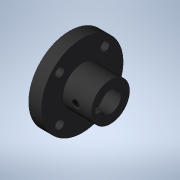
# Autodesk Inventor part: STHRANG8-MB_ss
Saved by Autodesk Inventor 2021 (Build 250183000, 183)
## iProperties
Created: 2025-08-06
Part Number: STHRANG8-MB_ss
Material: Generic
Catalog Web Link: www.cadenas.de
Description: STHRBNG, STHRNG, SSTHRNG, STHRANG_SS-Shaft Supports - with Damper - Key Groove - Round Flange
Vendor: MISUMI
Document SubType Name: Modeling
Designer: psAdmin
Manufacturer: MISUMI
Mass: 4.85232 g
Surface Area: 31.4741 cm^2
Volume: 4.85232 cm^3
Density: 1 g/cm^3
Appearance: PSOLRGB-175-175-175
Category: PARTsolutions
Company: MISUMI
Title: STHRANG8-MB
Author: Cadenas PARTsolutions
Comments: Shaft Supports - with Damper - Key Groove - Round Flange
PSOL_IDENT_0: {$CADENAS_DATA/23d-libs/misumi/metric/02_shaft_supports/sthrbng/sthrbng.prj},207 {VTYP=3D},{NB=STHRA
PSOL_IDENT_1: NG8-MB_ss},{LINA=STHRANG8-MB},{NN=STHRBNG, STHRNG, SSTHRNG, STHRANG_SS},{DATE=18.02.2024 15:03:40},{
PSOL_IDENT_2: GEOMDATE=16.02.2024 10:05:26},{VERSION=},{LINEID=190},{WBVAR=MAT,ST,ALT1},{WBNUMERIC=}  {NB=STHRANG8
PSOL_IDENT_3: -MB_ss},{LINA=STHRANG8-MB},{KT=DUMMY},{PN=STHRANG8-MB},{TYPE=STHRANG},{MAT=5052},{ST=-},{D=8},{DTOL=
PSOL_IDENT_4: +0.015/0},{N=3.5},{L=16},{S=0},{L1=0},{D1=15},{H=32},{T=5},{LL=10},{M=M3},{THMD=3},{THDMIN=2.459},{P=
PSOL_IDENT_5: 25},{K=0},{W=15},{P1=25},{F=0},{DD1=3.5},{ST0='-','-'},{BB=3},{BBTOL=+0.013/-0.013},{TT=1.8},{TTTOL=
PSOL_IDENT_6: +0.1/0},{ALT1=MB},{MBM=M3},{ML=3},{ALT1PN=-MB},{MATALG= '1045', 'S45C Equivalent', '304', 'SUS304','
PSOL_IDENT_7: 5052','5052 Aluminum Alloy' }
NB: STHRANG8-MB_ss
NN: STHRBNG, STHRNG, SSTHRNG, STHRANG_SS
NT: Shaft Supports - with Damper - Key Groove - Round Flange
NBSYN: $PN._ss
LINA: STHRANG8-MB
CATALOG: Misumi
PN: STHRANG8-MB
MAT: 5052 Aluminum Alloy
ST: -
D: 8
DTOL: +0.015/0
N: 3.5
L: 16
S: 0
L1: 0
D1: 15
H: 32
T: 5
LL: 10
M: M3
P: 25
W: 15
P1: 25
F: 0
DD1: 3.5
BB: 3
BBTOL: +0.013/-0.013
TT: 1.8
TTTOL: +0.1/0
MBM: M3
ML: 3
SUPPLIER: MISUMI
ARTICLENO: STHRANG8-MB_ss
BOMINFO: STHRANG8-MB
CREATOR: CADENAS GmbH
Autodesk Inventor part; units mm, degrees
sketch "Sketch_1" plane through (0, 0, 0) normal (0, 0, 1) x (1, 0, 0)
  line L0 (16, 0) -> (0, 0)
  line L1 (0, 4) -> (16, 4)
  line L2 (16, 4) -> (16, 7.5)
  line L3 (16, 7.5) -> (5, 7.5)
  line L4 (5, 7.5) -> (5, 16)
  line L5 (5, 16) -> (0, 16)
  line L6 (0, 16) -> (0, 4)
  constraints: 14 end point
revolve "Revolution1" add sketch "Sketch_1" angle 360 about axis through (16, 0, 0) along (1, 0, 0)
sketch "Sketch2" plane through (0, 0, 0) normal (-1, 0, 0) x (0, 0, 1)
  point P0 (-8.8388, 8.8388)
hole "Hole1" at (0, 8.8388, -8.8388) direction (1, 0, 0) diameter 3.5 depth 5
pattern_linear "Rectangular Pattern1" count 2 spacing 17.6777 along (0, 0, 1) count 2 spacing 17.6777 along (0, -1, 0) of "Hole1"
sketch "Sketch_4" plane through (10, 0, 0) normal (1, 0, 0) x (0, 0, -1)
  line L0 (0, -7.5) -> (0, -3)
  line L1 (0, -3) -> (1.2295, -3)
  line L2 (1.2295, -3) -> (1.2295, -7.2295)
  line L3 (1.2295, -7.2295) -> (1.5, -7.5)
  line L4 (1.5, -7.5) -> (0, -7.5)
  line L5 (0, -7.5) -> (0, -3)
  constraints: 12 end point
revolve "Revolution2" cut sketch "Sketch_4" angle 360 about axis through (10, -7.5, 0) along (0, -1, 0)
thread "Thread1" size "M3x0.5" class "6H" standard "ISO Metric profile" length 3.2295
sketch "Sketch_8" plane through (0, 0, 0) normal (1, 0, 0) x (0, 1, 0)
  line L0 (1.5, 5.8) -> (-1.5, 5.8)
  line L1 (-1.5, 5.8) -> (-1.5, 0)
  line L2 (-1.5, 0) -> (1.5, 0)
  line L3 (1.5, 0) -> (1.5, 5.8)
  constraints: 8 end point
extrude "Extrusion1" cut sketch "Sketch_8" along normal blind 16
sketch "Sketch_5" plane through (10, 0, 0) normal (1, 0, 0) x (0, 0, -1)
  line L0 (-4, 0) -> (-7.5, 0)
  line L1 (-7.5, 0) -> (-7.5, 1.5)
  line L2 (-7.5, 1.5) -> (-7.2295, 1.2295)
  line L3 (-7.2295, 1.2295) -> (-4, 1.2295)
  line L4 (-4, 1.2295) -> (-4, 0)
  line L5 (-4, 0) -> (-7.5, 0)
  constraints: 12 end point
revolve "Revolution3" cut sketch "Sketch_5" angle 360 about axis through (10, 0, 4) along (0, 0, -1)
thread "Thread2" size "M3x0.5" class "6H" standard "ISO Metric profile" length 1.4295
ref_plane "to_screw1_XY" through (10, 0, 5.8) normal (0, 0, 1) x (1, 0, 0)
ref_plane "to_screw1_YZ" through (10, 0, 5.8) normal (1, 0, 0) x (0, 1, 0)
ref_plane "to_screw1_ZX" through (10, 0, 5.8) normal (0, 1, 0) x (0, 0, 1)
ref_plane "to_screw2_XY" through (10, -4, 0) normal (0, -1, 0) x (1, 0, 0)
ref_plane "to_screw2_YZ" through (10, -4, 0) normal (1, 0, 0) x (0, 0, 1)
ref_plane "to_screw2_ZX" through (10, -4, 0) normal (0, 0, 1) x (0, -1, 0)
body "Solid1"
